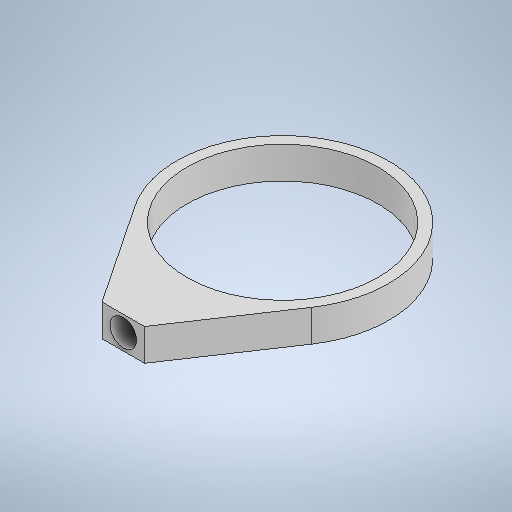
# Autodesk Inventor part: 21
Saved by Autodesk Inventor 2025.1 (Build 291241000, 241)
## iProperties
Created: 2024-09-13
Part Number: 21
Material: Generisch
Document SubType Name: Modeling
Designer: ffogue
Density: 1 g/cm^3
Appearance: Vorgabe
Author: ffogue
Autodesk Inventor part; units mm, degrees
ref_plane "YZ Plane" through (0, 0, 0) normal (1, 0, 0) x (0, 1, 0)
ref_plane "XZ Plane" through (0, 0, 0) normal (0, 1, 0) x (-1, 0, 0)
ref_plane "XY Plane" through (0, 0, 0) normal (0, 0, 1) x (1, 0, 0)
sketch "Sketch1" plane through (0, 0, 0) normal (0, 0, 1) x (1, 0, 0)
  line L0 (-2, 0) -> (2, 0)
  arc A0 (8.313, 9.4417) -> (-8.313, 9.4417) centre (0, 15) ccw
  line L1 (-2, 0) -> (-8.313, 9.4417)
  line L2 (2, 0) -> (8.313, 9.4417)
  line L3 (0, 0) -> (0, 7.2801) construction
  point P0 (0, 3.6401)
  dimension "d0" = 20
  dimension "d1" = 4
  dimension "d2" = 15
  constraints: 8 end point, 2 horizontal alignment, 2 midpoint, 2 point on circle, 1 centre point, 1 coincident, 1 horizontal, 1 symmetric about line, 1 tangent, 1 vertical, 1 vertical alignment
  measures "d0" diameter of A0
  measures "d1" distance of L0.start L0.end
  measures "d2" distance from line of A0.centre L0
extrude "Extrusion1" add sketch "Sketch1" along normal mid plane 3
sketch "Sketch2" plane through (0, 0, 1.5) normal (0, 0, 1) x (1, 0, 0)
  circle A0 centre (0, 15) radius 9
  arc A1 (8.313, 9.4417) -> (-8.313, 9.4417) centre (0, 15) ccw projected
  point P0 (0, 0)
  dimension "d5" = 18
  constraints: 1 centre point, 1 concentric
  measures "d5" diameter of A0
extrude "Extrusion2" cut sketch "Sketch2" against normal blind 3
sketch "Sketch3" plane through (-2, 0, 1.5) normal (0, -1, 0) x (1, 0, 0)
  circle A0 centre (2, -1.5) radius 1.25
  dimension "d8" = 2.5
  constraints: 1 centre point, 1 coincident
  measures "d8" diameter of A0
extrude "Extrusion3" cut sketch "Sketch3" against normal up to surface
body "Solid1"
